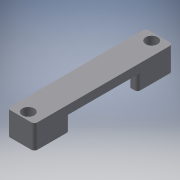
# Autodesk Inventor part: SyringeServoClamp
Saved by Autodesk Inventor 2018 (Build 220112000, 112)
## iProperties
Created: 2018-05-08
Part Number: SyringeServoClamp
Material: Generic
Document SubType Name: Modeling
Designer: reide
Density: 1 g/cm^3
Appearance: Default
Author: reide
Autodesk Inventor part; units mm, degrees
ref_plane "YZ Plane" through (0, 0, 0) normal (1, 0, 0) x (0, 1, 0)
ref_plane "XZ Plane" through (0, 0, 0) normal (0, 1, 0) x (-1, 0, 0)
sketch "Sketch1" plane through (0, 0, 0) normal (0, 0, 1) x (1, 0, 0)
  arc A0 (-3.52, 5.9525) -> (-4.52, 4.9525) centre (-3.52, 4.9525) ccw projected
  line L0 (-4.52, -4.8041) -> (-4.52, 4.9525) projected
  arc A1 (-4.52, -4.8041) -> (-3.52, -5.8041) centre (-3.52, -4.8041) ccw projected
  line L1 (-2.52, -5.8041) -> (-3.52, -5.8041) projected
  arc A2 (-2.52, -5.8041) -> (-1.52, -4.8041) centre (-2.52, -4.8041) ccw projected
  line L2 (-1.52, 0.9525) -> (-1.52, -4.8041) projected
  line L3 (1.52, 0.9525) -> (-1.52, 0.9525) projected
  line L4 (1.52, -4.8041) -> (1.52, 0.9525) projected
  arc A3 (1.52, -4.8041) -> (2.52, -5.8041) centre (2.52, -4.8041) ccw projected
  line L5 (3.52, -5.8041) -> (2.52, -5.8041) projected
  arc A4 (3.52, -5.8041) -> (4.52, -4.8041) centre (3.52, -4.8041) ccw projected
  line L6 (4.52, 4.9525) -> (4.52, -4.8041) projected
  arc A5 (4.52, 4.9525) -> (3.52, 5.9525) centre (3.52, 4.9525) ccw projected
  line L7 (-3.52, 5.9525) -> (3.52, 5.9525) projected
  arc A6 (2.52, -28.2909) -> (1.52, -29.2909) centre (2.52, -29.2909) ccw projected
  line L8 (1.52, -35.0475) -> (1.52, -29.2909) projected
  line L9 (-1.52, -35.0475) -> (1.52, -35.0475) projected
  line L10 (-1.52, -29.2909) -> (-1.52, -35.0475) projected
  arc A7 (-1.52, -29.2909) -> (-2.52, -28.2909) centre (-2.52, -29.2909) ccw projected
  line L11 (-3.52, -28.2909) -> (-2.52, -28.2909) projected
  arc A8 (-3.52, -28.2909) -> (-4.52, -29.2909) centre (-3.52, -29.2909) ccw projected
  line L12 (-4.52, -39.0475) -> (-4.52, -29.2909) projected
  arc A9 (-4.52, -39.0475) -> (-3.52, -40.0475) centre (-3.52, -39.0475) ccw projected
  line L13 (3.52, -40.0475) -> (-3.52, -40.0475) projected
  arc A10 (3.52, -40.0475) -> (4.52, -39.0475) centre (3.52, -39.0475) ccw projected
  line L14 (4.52, -29.2909) -> (4.52, -39.0475) projected
  arc A11 (4.52, -29.2909) -> (3.52, -28.2909) centre (3.52, -29.2909) ccw projected
  line L15 (2.52, -28.2909) -> (3.52, -28.2909) projected
  point P0 (0, 0)
extrude "Extrusion1" add sketch "Sketch1" along normal blind 5
sketch "Sketch2" plane through (0, 0, 5) normal (0, 0, 1) x (1, 0, 0)
  arc A0 (-3.52, 5.9525) -> (-4.52, 4.9525) centre (-3.52, 4.9525) ccw projected
  line L0 (-4.52, 4.9525) -> (-4.52, -4.8041) projected
  arc A1 (-4.52, -4.8041) -> (-3.52, -5.8041) centre (-3.52, -4.8041) ccw projected
  line L1 (-3.52, -5.8041) -> (-2.52, -5.8041) projected
  arc A2 (-2.52, -5.8041) -> (-1.52, -4.8041) centre (-2.52, -4.8041) ccw projected
  line L2 (-1.52, -4.8041) -> (-1.52, 0.9525) projected
  line L3 (-1.52, 0.9525) -> (1.52, 0.9525) projected
  line L4 (1.52, 0.9525) -> (1.52, -4.8041) projected
  arc A3 (1.52, -4.8041) -> (2.52, -5.8041) centre (2.52, -4.8041) ccw projected
  line L5 (2.52, -5.8041) -> (3.52, -5.8041) projected
  arc A4 (3.52, -5.8041) -> (4.52, -4.8041) centre (3.52, -4.8041) ccw projected
  line L6 (4.52, -4.8041) -> (4.52, 4.9525) projected
  arc A5 (4.52, 4.9525) -> (3.52, 5.9525) centre (3.52, 4.9525) ccw projected
  line L7 (3.52, 5.9525) -> (-3.52, 5.9525) projected
  arc A6 (2.52, -28.2909) -> (1.52, -29.2909) centre (2.52, -29.2909) ccw projected
  line L8 (1.52, -29.2909) -> (1.52, -35.0475) projected
  line L9 (1.52, -35.0475) -> (-1.52, -35.0475) projected
  line L10 (-1.52, -35.0475) -> (-1.52, -29.2909) projected
  arc A7 (-1.52, -29.2909) -> (-2.52, -28.2909) centre (-2.52, -29.2909) ccw projected
  line L11 (-2.52, -28.2909) -> (-3.52, -28.2909) projected
  arc A8 (-3.52, -28.2909) -> (-4.52, -29.2909) centre (-3.52, -29.2909) ccw projected
  line L12 (-4.52, -29.2909) -> (-4.52, -39.0475) projected
  arc A9 (-4.52, -39.0475) -> (-3.52, -40.0475) centre (-3.52, -39.0475) ccw projected
  line L13 (-3.52, -40.0475) -> (3.52, -40.0475) projected
  arc A10 (3.52, -40.0475) -> (4.52, -39.0475) centre (3.52, -39.0475) ccw projected
  line L14 (4.52, -39.0475) -> (4.52, -29.2909) projected
  arc A11 (4.52, -29.2909) -> (3.52, -28.2909) centre (3.52, -29.2909) ccw projected
  line L15 (3.52, -28.2909) -> (2.52, -28.2909) projected
  line L16 (-4.52, -4.8041) -> (4.52, -4.8041)
  line L17 (4.52, -4.8041) -> (4.52, -29.2909)
  line L18 (4.52, -29.2909) -> (-4.52, -29.2909)
  line L19 (-4.52, -29.2909) -> (-4.52, -4.8041)
  line L20 (-1.52, -35.0475) -> (1.52, -35.0475)
  line L21 (1.52, -35.0475) -> (1.52, 0.9525)
  line L22 (1.52, 0.9525) -> (-1.52, 0.9525)
  line L23 (-1.52, 0.9525) -> (-1.52, -35.0475)
  point P0 (0, 0)
  constraints: 16 end point, 4 parallel, 2 horizontal, 2 perpendicular
ref_plane "Work Plane1" through (-13.8343, -45.838, 7.888) normal (0, 0, -1) x (0, 1, 0)
extrude "Extrusion2" add sketch "Sketch2" along normal up to surface (2.888 mm away)
sketch "Sketch3" plane through (-3.52, 5.9525, 7.888) normal (0, 0, 1) x (1, 0, 0)
  arc A0 (6.04, -34.2434) -> (5.04, -35.2434) centre (6.04, -35.2434) ccw projected
  line L0 (5.04, -41) -> (5.04, -35.2434) projected
  line L1 (2, -41) -> (5.04, -41) projected
  line L2 (2, -35.2434) -> (2, -41) projected
  arc A1 (2, -35.2434) -> (1, -34.2434) centre (1, -35.2434) ccw projected
  line L3 (0, -34.2434) -> (1, -34.2434) projected
  arc A2 (0, -34.2434) -> (-1, -35.2434) centre (0, -35.2434) ccw projected
  line L4 (-1, -45) -> (-1, -35.2434) projected
  arc A3 (-1, -45) -> (0, -46) centre (0, -45) ccw projected
  line L5 (7.04, -46) -> (0, -46) projected
  arc A4 (7.04, -46) -> (8.04, -45) centre (7.04, -45) ccw projected
  line L6 (8.04, -35.2434) -> (8.04, -45) projected
  arc A5 (8.04, -35.2434) -> (7.04, -34.2434) centre (7.04, -35.2434) ccw projected
  line L7 (6.04, -34.2434) -> (7.04, -34.2434) projected
  arc A6 (0, 0) -> (-1, -1) centre (0, -1) ccw projected
  line L8 (-1, -10.7566) -> (-1, -1) projected
  arc A7 (-1, -10.7566) -> (0, -11.7566) centre (0, -10.7566) ccw projected
  line L9 (1, -11.7566) -> (0, -11.7566) projected
  arc A8 (1, -11.7566) -> (2, -10.7566) centre (1, -10.7566) ccw projected
  line L10 (2, -5) -> (2, -10.7566) projected
  line L11 (5.04, -5) -> (2, -5) projected
  line L12 (5.04, -10.7566) -> (5.04, -5) projected
  arc A9 (5.04, -10.7566) -> (6.04, -11.7566) centre (6.04, -10.7566) ccw projected
  line L13 (7.04, -11.7566) -> (6.04, -11.7566) projected
  arc A10 (7.04, -11.7566) -> (8.04, -10.7566) centre (7.04, -10.7566) ccw projected
  line L14 (8.04, -1) -> (8.04, -10.7566) projected
  arc A11 (8.04, -1) -> (7.04, 0) centre (7.04, -1) ccw projected
  line L15 (0, 0) -> (7.04, 0) projected
  line L16 (0, -46) -> (7.04, -46) projected
  line L17 (3.52, -46) -> (3.52, -41)
  line L18 (2, -41) -> (5.04, -41) projected
  circle A12 centre (3.52, -43.5) radius 1.375
  circle A13 centre (3.52, -43.5) radius 1.375
  line L19 (-1, -1) -> (-1, -45) projected
  line L20 (-1, -23) -> (-5.6453, -23)
  arc A14 (5.04, -10.7566) -> (6.04, -11.7566) centre (6.04, -10.7566) ccw
  line L21 (5.04, -5) -> (5.04, -10.7566)
  line L22 (2, -5) -> (5.04, -5)
  line L23 (2, -10.7566) -> (2, -5)
  arc A15 (1, -11.7566) -> (2, -10.7566) centre (1, -10.7566) ccw
  line L24 (0, -11.7566) -> (1, -11.7566)
  arc A16 (-1, -10.7566) -> (0, -11.7566) centre (0, -10.7566) ccw
  line L25 (-1, -1) -> (-1, -10.7566)
  arc A17 (0, 0) -> (-1, -1) centre (0, -1) ccw
  line L26 (7.04, 0) -> (0, 0)
  arc A18 (8.04, -1) -> (7.04, 0) centre (7.04, -1) ccw
  line L27 (8.04, -10.7566) -> (8.04, -1)
  arc A19 (7.04, -11.7566) -> (8.04, -10.7566) centre (7.04, -10.7566) ccw
  line L28 (6.04, -11.7566) -> (7.04, -11.7566)
  line L29 (0, 0) -> (7.04, 0)
  line L30 (3.52, 0) -> (3.52, -5)
  line L31 (2, -5) -> (5.04, -5)
  circle A20 centre (3.52, -2.5) radius 1.375
  circle A21 centre (3.52, -2.5) radius 1.375
  line L32 (-1, -45) -> (-1, -1)
  point P0 (3.52, -5.9525)
  dimension "d5" = 2.75
  dimension "d6" = 2.75
  constraints: 28 end point, 13 symmetric about line, 12 point on circle, 10 centre point, 4 coincident, 4 midpoint, 1 horizontal, 8 other
  measures "d5" diameter of A12
  measures "d6" diameter of A13
extrude "Extrusion3" cut sketch "Sketch3" against normal blind 100 contours A12 L17 | L17 A12 | A20 L30 | L30 A20
body "Solid1"
